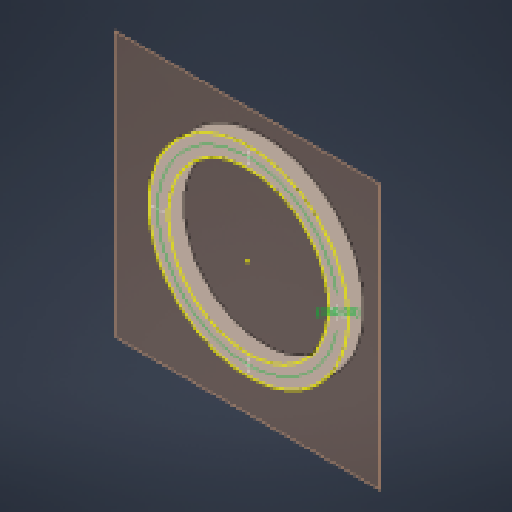
# Autodesk Inventor part: IR
Saved by Autodesk Inventor 2024 (Build 280153000, 153)
## iProperties
Created: 2023-10-21
Part Number: IR
Material: Generic
Document SubType Name: Modeling
Designer: range
Density: 1 g/cm^3
Appearance: Default
Author: range
Autodesk Inventor part; units mm, degrees
ref_plane "YZ Plane" through (0, 0, 0) normal (1, 0, 0) x (0, 1, 0)
ref_plane "XZ Plane" through (0, 0, 0) normal (0, 1, 0) x (-1, 0, 0)
ref_plane "Work Plane1" through (0, 0, 0) normal (0, 0, 1) x (1, 0, 0)
sketch "Sketch1" plane through (0, 0, 0) normal (0, 0, 1) x (1, 0, 0)
  circle A0 centre (0, 0) radius 62.3 projected
  circle A1 centre (0, 0) radius 49.5
  circle A2 centre (0, 0) radius 61.5
  line L0 (49.5, 0) -> (61.5, 0) construction
  point P0 (55.5, 0)
  point P1 (0, 55.5)
  point P2 (-55.5, 0)
  point P3 (0, -55.5)
  dimension "d0" = 99
  dimension "d1" = 12
  dimension "d4" = 360
  constraints: 2 end point, 2 horizontal alignment, 1 coincident, 1 horizontal, 1 midpoint, 1 point on line, 9 other
ref_plane "Work Plane2" through (-74.3, -74.3, -10) normal (0, 0, -1) x (0, 1, 0)
extrude "Extrusion1" add sketch "Sketch1" against normal up to surface (10 mm away) contours A2
sketch "Sketch2" plane through (0, 0, 0) normal (0, 0, 1) x (1, 0, 0)
  circle A0 centre (0, 0) radius 49.5 projected
  line L0 (49.5, 0) -> (61.5, 0) construction
  circle A1 centre (0, 0) radius 61.5 projected
  point P0 (55.5, 0)
  point P1 (0, 55.5)
  point P2 (-55.5, 0)
  point P3 (0, -55.5)
  dimension "d10" = 360
  constraints: 2 end point, 2 horizontal alignment, 1 horizontal, 1 midpoint, 1 point on line, 7 other
hole "Hole1" at (55.5, 0, 0) at (0, 55.5, 0) at (-55.5, 0, 0) at (0, -55.5, 0) direction (0, 0, -1) diameter 5 end through all countersink diameter 10.3886 countersink angle 90 clearance for "Flat Head Machine Screw" size "M5" standard "Ansi Metric M Profile"
body "Solid1"
